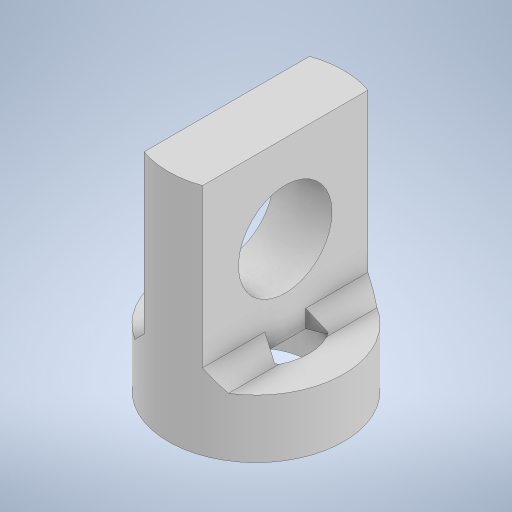
# Autodesk Inventor part: anchor_end_3.0mm_new
Saved by Autodesk Inventor 2024 (Build 280153000, 153)
## iProperties
Created: 2024-06-07
Part Number: anchor_end_3.0mm_new
Material: 일반
Document SubType Name: Modeling
Designer: Gihyeok Na
Density: 1 g/cm^3
Appearance: 기본값
Author: Gihyeok Na
Autodesk Inventor part; units mm, degrees
ref_plane "YZ Plane" through (0, 0, 0) normal (1, 0, 0) x (0, 1, 0)
ref_plane "XZ Plane" through (0, 0, 0) normal (0, 1, 0) x (-1, 0, 0)
ref_plane "XY Plane" through (0, 0, 0) normal (0, 0, 1) x (1, 0, 0)
sketch "스케치2" plane through (0, 0, 0) normal (0, 1, 0) x (-1, 0, 0)
  circle A0 centre (0, 0) radius 1.5
  circle A1 centre (0, 0) radius 0.9
  dimension "d0" = 3
  dimension "d6" = 1.8
  constraints: 2 centre point, 2 coincident
  measures "d0" diameter of A0
  measures "d6" diameter of A1
extrude "돌출1" add sketch "스케치2" along normal blind 1
sketch "스케치4" plane through (0, 1, 0) normal (0, 1, 0) x (1, 0, 0)
  line L0 (0.5, -1.55) -> (-0.5, -1.55)
  line L1 (-0.5, -1.55) -> (-0.5, 1.55)
  line L2 (-0.5, 1.55) -> (0.5, 1.55)
  line L3 (0.5, 1.55) -> (0.5, -1.55)
  line L4 (0.5, -1.55) -> (-0.5, 1.55) construction
  line L5 (-0.5, -1.55) -> (0.5, 1.55) construction
  circle A0 centre (0, 0) radius 1.5 projected
  point P0 (0.5, 1.4142)
  point P1 (-0.5, 1.4142)
  point P2 (-0.5, -1.4142)
  point P3 (0.5, -1.4142)
  dimension "d7" = 1
  constraints: 12 end point, 2 midpoint, 2 parallel, 1 horizontal, 1 perpendicular
  measures "d7" distance of L1.end L2.end
extrude "돌출3" add sketch "스케치4" along normal blind 3 contours A0 L1 L3
chamfer "모따기1" distance 0.3 angle 45 4 edges at (0.5, 1, -1.0813) (0.5, 1, 1.0813) (-0.5, 1, -1.0813) (-0.5, 1, 1.0813)
chamfer "모따기2" distance 0.4 angle 45 4 edges at (-0.5, 1.15, -0.7483) (0.5, 1.15, -0.7483) (0.5, 1.15, 0.7483) (-0.5, 1.15, 0.7483)
sketch "스케치5" plane through (0.5, 4, 1.4142) normal (1, 0, 0) x (0, 0, -1)
  line L0 (1.0659, -3) -> (1.0659, -2.7) projected
  line L1 (1.0659, -3) -> (1.7625, -3) projected
  line L2 (1.7625, -2.7) -> (1.7625, -3) projected
  line L3 (2.8284, -2.7) -> (1.7625, -2.7) projected
  line L4 (2.8284, -2.7) -> (2.8284, 0) projected
  line L5 (0, 0) -> (2.8284, 0) projected
  line L6 (0, -2.7) -> (0, 0) projected
  line L7 (1.0659, -2.7) -> (0, -2.7) projected
  circle A0 centre (1.4142, -1.5) radius 0.8
  point P0 (1.4142, -4)
  dimension "d16" = 1.6
  dimension "d17" = 1.5
  constraints: 1 centre point
  measures "d16" diameter of A0
  measures "d17" distance from line of A0.centre L5
extrude "돌출4" cut sketch "스케치5" against normal blind 3 contours A0
